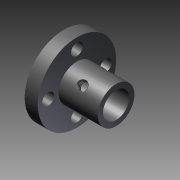
# Autodesk Inventor part: STHRB10M-MB_b
Saved by Autodesk Inventor 2011 SP1 (Build 150282100, 282)
## iProperties
Created: 2016-06-28
Part Number: STHRB10M-MB_b
Catalog Web Link: www.cadenas.de
Description: STHRB, STHR, SSTHR, ATHR, BTHR_b-Shaft Supports - Bracket Shaped - Standard Drilled Mounting Hole Type - Round Flange
Vendor: MISUMI
Document SubType Name: Modeling
Designer: psAdmin
Manufacturer: MISUMI
Mass: 3.92034 g
Surface Area: 31.7611 cm^2
Volume: 3.92034 cm^3
Density: 1 g/cm^3
Category: PARTsolutions
Company: MISUMI
Title: STHRB10M-MB
Author: Cadenas PARTsolutions
Comments: Shaft Supports - Bracket Shaped - Standard Drilled Mounting Hole Type - Round Flange
PSOL_IDENT_0: {$CADENAS_DATA\23d-libs\misumi\metric\02_shaft_supports\ssthr\ssthr_body.prj},204 {VTYP=3D},{NB=STHR
PSOL_IDENT_1: B10M-MB_b},{LINA=STHRB10M-MB},{NN=STHRB, STHR, SSTHR, ATHR, BTHR_b},{DATE=26.05.2016 07:04:25},{GEOM
PSOL_IDENT_2: DATE=06.10.2015 08:50:00},{VERSION=},{LINEID=60},{LINESUBID=-1},{WBVAR=MAT,ST,M,ALT}  {NB=STHRB10M-M
PSOL_IDENT_3: B_b},{LINA=STHRB10M-MB},{KT=DUMMY},{PN=STHRB10M-MB},{TS=1},{TSALG= '1', 'Drilled Mounting Hole', '2'
PSOL_IDENT_4: , 'Tapped Mounting Hole' },{TYPE=STHRB},{MAT=1018},{MATA= '1018', 'SS400 Equivalent', '304', 'SUS304'
PSOL_IDENT_5: , 'AA'  , 'Aluminum Alloy' },{MALG='M3','M4'},{ST=BO},{ST0= 'BO', 'Black Oxide', 'ENP', 'Electroless
PSOL_IDENT_6: Nickel Plating' },{D=10},{THMD11='M3','M4'},{THMD13='M4'},{THMD12='M3'},{DTOL=+0.015/0},{DX=10},{N=
PSOL_IDENT_7: 2.0},{L=20},{D1=14},{H=30},{T=5.0},{LL=12},{M=M4},{THMD=4},{THMD1=M3,M4},{THMD2=M3,M4},{P=22},{K=23}
PSOL_IDENT_8: ,{W=18},{P1=22},{F=0},{DD1=4.5},{DD11=3.5,4.5},{DD12=3.5,4.5},{M1=M4},{M11=4},{ALT=MB},{ALTPN=-MB},{
PSOL_IDENT_9: BM=4.0},{BL=3.0}
NN: STHRB, STHR, SSTHR, ATHR, BTHR_b
NT: Shaft Supports - Bracket Shaped - Standard Drilled Mounting Hole Type - Round Flange
NB: STHRB10M-MB_b
NBSYN: $PN._b
LINA: STHRB10M-MB
PN: STHRB10M-MB
MAT: SS400 Equivalent
ST: Black Oxide
D: 10
DTOL: +0.015/0
N: 2.0
L: 20
D1: 14
H: 30
T: 5.0
LL: 12
M: M4
P: 22
DD1: 4.5
ALT: with MB (Hex Socket Set Screw Included)
SUPPLIER: MISUMI
ARTICLENO: STHRB10M-MB_b
BOMINFO: STHRB10M-MB
CREATOR: CADENAS GmbH
Autodesk Inventor part; units mm, degrees
ref_plane "YZ Plane" through (0, 0, 0) normal (1, 0, 0) x (0, 1, 0)
ref_plane "XZ Plane" through (0, 0, 0) normal (0, 1, 0) x (-1, 0, 0)
ref_plane "XY Plane" through (0, 0, 0) normal (0, 0, 1) x (1, 0, 0)
sketch "Sketch_1" plane through (0, 0, 0) normal (0, 0, 1) x (1, 0, 0)
  line L0 (20, 0) -> (0, 0)
  line L1 (0, 15) -> (0, 5)
  line L2 (0, 5) -> (20, 5)
  line L3 (20, 5) -> (20, 7)
  line L4 (20, 7) -> (5, 7)
  line L5 (5, 7) -> (5, 15)
  line L6 (5, 15) -> (0, 15)
  constraints: 14 end point
revolve "Revolution1" add sketch "Sketch_1" angle 360 about axis through (20, 0, 0) along (1, 0, 0)
sketch "Sketch_3" plane through (0, 0, 0) normal (0, -0.7071068, 0.7071068) x (1, 0, 0)
  line L0 (12, 4.5) -> (12, 7)
  line L1 (12, 7) -> (14, 7)
  line L2 (14, 7) -> (13.621, 6.621)
  line L3 (13.621, 6.621) -> (13.621, 4.5)
  line L4 (13.621, 4.5) -> (12, 4.5)
  line L5 (12, 4.5) -> (12, 7)
  constraints: 12 end point
revolve "Revolution2" cut sketch "Sketch_3" angle 360 about axis through (12, 3.182, 3.182) along (0, -0.7071068, -0.7071068)
thread "Thread1" size "M4x0.7" class "6H" standard "ISO Metric profile" length 2.121
sketch "Sketch3" plane through (5, 0, 0) normal (1, 0, 0) x (0, 0, -1)
  point P0 (0, 11)
hole "Hole1" at (5, 11, 0) direction (-1, 0, 0) diameter 4.5 depth 5
sketch "Sketch4" plane through (5, 0, 0) normal (1, 0, 0) x (0, 0, -1)
  point P0 (0, -11)
hole "Hole2" at (5, -11, 0) direction (-1, 0, 0) diameter 4.5 depth 5
sketch "Sketch5" plane through (5, 0, 0) normal (1, 0, 0) x (0, 0, -1)
  point P0 (-11, 0)
hole "Hole3" at (5, 0, 11) direction (-1, 0, 0) diameter 4.5 depth 5
sketch "Sketch6" plane through (5, 0, 0) normal (1, 0, 0) x (0, 0, -1)
  point P0 (11, 0)
hole "Hole4" at (5, 0, -11) direction (-1, 0, 0) diameter 4.5 depth 5
sketch "Sketch_2" plane through (0, 0, 0) normal (0, -0.7071068, -0.7071068) x (1, 0, 0)
  line L0 (12, 4.5) -> (12, 7)
  line L1 (12, 7) -> (14, 7)
  line L2 (14, 7) -> (13.621, 6.621)
  line L3 (13.621, 6.621) -> (13.621, 4.5)
  line L4 (13.621, 4.5) -> (12, 4.5)
  line L5 (12, 4.5) -> (12, 7)
  constraints: 12 end point
revolve "Revolution3" cut sketch "Sketch_2" angle 360 about axis through (12, -3.182, 3.182) along (0, 0.7071068, -0.7071068)
thread "Thread2" size "M4x0.7" class "6H" standard "ISO Metric profile" length 2.121
ref_plane "to_screw1_XY" through (12, 3.5355, 3.5355) normal (0, 0.7071068, 0.7071068) x (1, 0, 0)
ref_plane "to_screw1_YZ" through (12, 3.5355, 3.5355) normal (1, 0, 0) x (0, 0.7071068, -0.7071068)
ref_plane "to_screw1_ZX" through (12, 3.5355, 3.5355) normal (0, 0.7071068, -0.7071068) x (0, 0.7071068, 0.7071068)
ref_plane "to_screw2_XY" through (12, -3.5355, 3.5355) normal (0, -0.7071068, 0.7071068) x (1, 0, 0)
ref_plane "to_screw2_YZ" through (12, -3.5355, 3.5355) normal (1, 0, 0) x (0, 0.7071068, 0.7071068)
ref_plane "to_screw2_ZX" through (12, -3.5355, 3.5355) normal (0, 0.7071068, 0.7071068) x (0, -0.7071068, 0.7071068)
body "Solid1"
